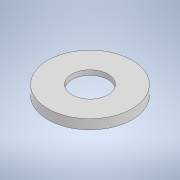
# Autodesk Inventor part: Корпус дросселя
Saved by Autodesk Inventor 2021 (Build 250183000, 183)
## iProperties
Created: 2020-11-05
Part Number: Корпус дросселя
Material: Типовые
Document SubType Name: Modeling
Designer: Тимоха
Density: 1 g/cm^3
Appearance: По умолчанию
Author: Тимоха
Autodesk Inventor part; units mm, degrees
ref_plane "YZ Plane" through (0, 0, 0) normal (1, 0, 0) x (0, 1, 0)
ref_plane "XZ Plane" through (0, 0, 0) normal (0, 1, 0) x (-1, 0, 0)
ref_plane "XY Plane" through (0, 0, 0) normal (0, 0, 1) x (1, 0, 0)
sketch "Эскиз1" plane through (0, 0, 0) normal (0, 0, 1) x (1, 0, 0)
  line L0 (0, 0) -> (0, 8)
  line L1 (0, 8) -> (0, 16)
  line L2 (0, 16) -> (70, 16)
  line L3 (70, 16) -> (70, 0)
  line L4 (70, 0) -> (50, 0)
  line L5 (50, 0) -> (50, 8)
  line L6 (50, 8) -> (30, 8)
  line L7 (30, 8) -> (30, 16)
  dimension "d0" = 8
  dimension "d1" = 8
  dimension "d2" = 70
  dimension "d3" = 20
  dimension "d4" = 20
  constraints: 16 end point, 5 perpendicular, 3 vertical, 1 point on line
  measures "d0" distance of L0.start L0.end
  measures "d1" distance of L0.end L1.end
  measures "d2" distance of L1.end L2.end
  measures "d3" distance of L3.end L4.end
  measures "d4" distance of L5.end L6.end
revolve "Вращение1" add sketch "Эскиз1" angle 360 about axis through (0, 8, 0) along (0, 1, 0)
